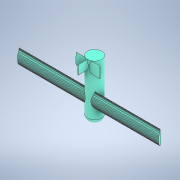
# Autodesk Inventor part: DimensionAccurateModel
Saved by Autodesk Inventor 2021 (Build 250183000, 183)
## iProperties
Created: 2021-11-10
Part Number: DimensionAccurateModel
Material: Generic
Document SubType Name: Modeling
Designer: PC
Density: 1 g/cm^3
Appearance: Default
Author: PC
Autodesk Inventor part; units mm, degrees
ref_plane "YZ Plane" through (0, 0, 0) normal (1, 0, 0) x (0, 1, 0)
ref_plane "XZ Plane" through (0, 0, 0) normal (0, 1, 0) x (-1, 0, 0)
ref_plane "XY Plane" through (0, 0, 0) normal (0, 0, 1) x (1, 0, 0)
sketch "Sketch1" plane through (0, 0, 0) normal (1, 0, 0) x (0, 1, 0)
  line L0 (-600.7431, 22.1358) -> (-593.9138, 28.6451)
  line L1 (-593.9138, 28.6451) -> (-585.2099, 34.8338)
  line L2 (-585.2099, 34.8338) -> (-574.687, 40.6463)
  line L3 (-574.687, 40.6463) -> (-562.4139, 46.1748)
  line L4 (-562.4139, 46.1748) -> (-548.4699, 51.3295)
  line L5 (-548.4699, 51.3295) -> (-532.9458, 56.0856)
  line L6 (-532.9458, 56.0856) -> (-515.9423, 60.404)
  line L7 (-515.9423, 60.404) -> (-497.5695, 64.272)
  line L8 (-497.5695, 64.272) -> (-477.9459, 67.6498)
  line L9 (-477.9459, 67.6498) -> (-457.2, 70.5082)
  line L10 (-457.2, 70.5082) -> (-435.4653, 72.8216)
  line L11 (-435.4653, 72.8216) -> (-412.8833, 74.5535)
  line L12 (-412.8833, 74.5535) -> (-389.6008, 75.6599)
  line L13 (-389.6008, 75.6599) -> (-365.7679, 76.0836)
  line L14 (-365.7679, 76.0836) -> (-341.5394, 75.7513)
  line L15 (-341.5394, 75.7513) -> (-317.0731, 74.5852)
  line L16 (-317.0731, 74.5852) -> (-292.5269, 72.493)
  line L17 (-292.5269, 72.493) -> (-268.0606, 69.3804)
  line L18 (-268.0606, 69.3804) -> (-243.8321, 65.1949)
  line L19 (-243.8321, 65.1949) -> (-219.9992, 59.9889)
  line L20 (-219.9992, 59.9889) -> (-196.7167, 53.9222)
  line L21 (-196.7167, 53.9222) -> (-174.1347, 47.2391)
  line L22 (-174.1347, 47.2391) -> (-152.4, 40.3738)
  line L23 (-152.4, 40.3738) -> (-131.6661, 33.8246)
  line L24 (-131.6661, 33.8246) -> (-112.0548, 28.0207)
  line L25 (-112.0548, 28.0207) -> (-93.6257, 23.2186)
  line L26 (-93.6257, 23.2186) -> (-76.6377, 18.7921)
  line L27 (-76.6377, 18.7921) -> (-61.1301, 15.1187)
  line L28 (-61.1301, 15.1187) -> (-47.2128, 12.0786)
  line L29 (-47.2128, 12.0786) -> (-34.913, 9.628)
  line L30 (-34.913, 9.628) -> (-24.3636, 7.3236)
  line L31 (-24.3636, 7.3236) -> (-15.6561, 5.0547)
  line L32 (-15.6561, 5.0547) -> (-8.8324, 3.0353)
  line L33 (-8.8324, 3.0353) -> (-3.8848, 1.571)
  line L34 (-3.8848, 1.571) -> (-0.9882, 0.3517)
  line L35 (-0.9882, 0.3517) -> (0, 0)
  line L36 (0, 0) -> (-0.9881, 0.0689)
  line L37 (-0.9881, 0.0689) -> (-3.9462, 0.2751)
  line L38 (-3.9462, 0.2751) -> (-8.8567, 0.5389)
  line L39 (-8.8567, 0.5389) -> (-15.6806, 0.9054)
  line L40 (-15.6806, 0.9054) -> (-24.3773, 1.3726)
  line L41 (-24.3773, 1.3726) -> (-34.9136, 1.5171)
  line L42 (-34.9136, 1.5171) -> (-47.1922, 1.2988)
  line L43 (-47.1922, 1.2988) -> (-61.1294, 0.6365)
  line L44 (-61.1294, 0.6365) -> (-76.6556, -0.1013)
  line L45 (-76.6556, -0.1013) -> (-93.6499, -1.4047)
  line L46 (-93.6499, -1.4047) -> (-112.0303, -2.8143)
  line L47 (-112.0303, -2.8143) -> (-131.6825, -4.3215)
  line L48 (-131.6825, -4.3215) -> (-152.4146, -6.5282)
  line L49 (-152.4146, -6.5282) -> (-174.1084, -8.8373)
  line L50 (-174.1084, -8.8373) -> (-196.6964, -10.5696)
  line L51 (-196.6964, -10.5696) -> (-220.0014, -11.6771)
  line L52 (-220.0014, -11.6771) -> (-243.8398, -12.81)
  line L53 (-243.8398, -12.81) -> (-268.064, -13.9611)
  line L54 (-268.064, -13.9611) -> (-292.5182, -15.1232)
  line L55 (-292.5182, -15.1232) -> (-317.0743, -15.5598)
  line L56 (-317.0743, -15.5598) -> (-341.5425, -15.9947)
  line L57 (-341.5425, -15.9947) -> (-365.7689, -16.4254)
  line L58 (-365.7689, -16.4254) -> (-389.5979, -16.849)
  line L59 (-389.5979, -16.849) -> (-428.3372, -16.3178)
  line L60 (-428.3372, -16.3178) -> (-435.4653, -16.4445)
  line L61 (-435.4653, -16.4445) -> (-457.1954, -15.8756)
  line L62 (-457.1954, -15.8756) -> (-477.9409, -15.3324)
  line L63 (-477.9409, -15.3324) -> (-497.5675, -14.8186)
  line L64 (-497.5675, -14.8186) -> (-515.9546, -14.3372)
  line L65 (-515.9546, -14.3372) -> (-532.9456, -12.9321)
  line L66 (-532.9456, -12.9321) -> (-548.4597, -11.6491)
  line L67 (-548.4597, -11.6491) -> (-562.411, -10.4953)
  line L68 (-562.411, -10.4953) -> (-574.7179, -9.4776)
  line L69 (-574.7179, -9.4776) -> (-585.2099, -7.6352)
  line L70 (-585.2099, -7.6352) -> (-593.9138, -6.1021)
  line L71 (-593.9138, -6.1021) -> (-600.7431, -4.5799)
  line L72 (-600.7431, -4.5799) -> (-605.6528, -3.0053)
  line L73 (-605.6528, -3.0053) -> (-608.6118, -1.2046)
  line L74 (-600.7431, 22.1358) -> (-605.6528, 15.9697)
  line L75 (-605.6528, 15.9697) -> (-608.0868, 11.3931)
  line L76 (-608.6118, -1.2046) -> (-609.6, 0)
  arc A0 (-608.0868, 11.3931) -> (-609.6, 0) centre (-597.4909, 4.1887) ccw
  point P0 (0, 0)
  point P1 (0, 0)
  constraints: 154 end point, 22 collinear, 16 parallel, 2 point on circle, 1 centre point, 1 coincident
extrude "Extrusion1" add sketch "Sketch1" along normal blind 6000
ref_plane "Work Plane1" through (3000, 0, 0) normal (1, 0, 0) x (0, 0, -1)
sketch "Sketch2" plane through (3000, 0, 0) normal (1, 0, 0) x (0, 0, -1)
  line L0 (509.6, -1238.9444) -> (-100, -1238.9444)
  line L1 (-100, -1238.9444) -> (-100, 1121.0556)
  line L2 (-100, 1121.0556) -> (509.6, 1121.0556)
  line L3 (509.6, 1121.0556) -> (509.6, -1238.9444)
  line L4 (-0.2751, -3.9462) -> (0, 0) projected
  line L5 (-75.7513, -341.5394) -> (-76.0836, -365.7679) projected
  line L6 (204.8, -1238.9444) -> (204.8, 1121.0556)
  point P0 (0, 0)
  dimension "d3" = 2360
  dimension "d4" = 609.6
  dimension "d6" = 100
  constraints: 10 end point, 2 midpoint, 2 parallel, 1 coincident, 1 horizontal, 1 perpendicular
  measures "d3" distance of L2.end L0.start
  measures "d4" distance of L1.end L2.end
  measures "d6" distance from line of point (0, 0) L1
revolve "Revolution1" add sketch "Sketch2" angle 360 about axis through (3000, -1238.9444, -204.8) along (0, 1, 0) contours L0 L1 L2 L6
fillet "Fillet1" radius 200 1 edges at (3000, -1238.9444, -509.6)
sketch "Sketch3" plane through (3000, 0, 0) normal (1, 0, 0) x (0, 0, -1)
  line L0 (509.6, 1121.0556) -> (-100, 1121.0556) projected
  line L1 (204.8, 1121.0556) -> (-490.73, 1121.0556)
  line L2 (-490.73, 1121.0556) -> (-490.73, 737.422)
  line L3 (-490.73, 737.422) -> (204.8, 737.422)
  line L4 (204.8, 737.422) -> (204.8, 1121.0556)
  line L5 (-100, -1038.9444) -> (-100, 1121.0556) projected
  point P0 (0, 0)
  dimension "d9" = 390.73
  constraints: 8 end point, 2 parallel, 1 horizontal, 1 midpoint, 1 perpendicular
  measures "d9" distance between parallel lines of L5 L2
ref_plane "Work Plane2" through (3000, -1038.9444, 100) normal (0, 0, 1) x (1, 0, 0)
sketch "Sketch4" plane through (3000, -1038.9444, 100) normal (0, 0, 1) x (1, 0, 0)
  line L0 (0, 2160) -> (0, 1776.3664) projected
  spline S0 degree 2 poles (0, 1776.3664) (-59.4168, 1857.3842) (0, 2160) knots 0 0 0 1 1 1
  spline S1 degree 2 poles (0, 1776.3664) (59.4168, 1857.3842) (0, 2160) knots 0 0 0 1 1 1
  point P0 (-3000, 1038.9444)
  point P1 (-27.1153, 1860.9486)
  point P2 (27.1153, 1860.9486)
  point P3 (30.7822, 1923.9864)
  point P4 (-30.7209, 1922.0644)
  constraints: 1 symmetric about line, 6 other
extrude "Extrusion2" add sketch "Sketch4" along normal blind 390.73
sketch "Sketch5" plane through (3000, 0, 0) normal (1, 0, 0) x (0, 0, -1)
  line L0 (509.6, 1121.0556) -> (-100, 1121.0556) projected
  line L1 (-100, 1121.0556) -> (-38, 1121.0556)
  line L2 (-38, 1121.0556) -> (-38, 640.8956)
  line L3 (-38, 640.8956) -> (-100, 640.8956)
  line L4 (-100, 640.8956) -> (-100, 1121.0556)
  spline S0 degree 2 poles (-69, 640.8956) (-117.7968, 773.1997) (-69, 1121.0556) knots 0 0 0 1 1 1
  line L5 (-69, 640.8956) -> (-69, 701.9711)
  spline S1 degree 2 poles (-69, 640.8956) (-20.2032, 773.1997) (-69, 1121.0556) knots 0 0 0 1 1 1
  point P0 (0, 0)
  point P1 (-92.0986, 774.5446)
  point P2 (-45.9014, 774.5446)
  dimension "d12" = 480.16
  dimension "d13" = 62
  constraints: 10 end point, 2 midpoint, 2 parallel, 1 horizontal, 1 perpendicular, 1 symmetric about line, 1 vertical, 6 other
  measures "d12" distance of L1.end L2.end
  measures "d13" distance between parallel lines of L4 L2
extrude "Extrusion3" add sketch "Sketch5" along normal mid plane 1000 contours S1 S0
equation "\"d10\" = d9"
body "Solid1"
